Ladengriff_v3 (Autodesk Fusion 360 design; units mm, degrees)
Autodesk Fusion 360 part; units mm, degrees
sketch "Skizze1" plane through (0, 0, 0) normal (0, 1, 0) x (1, 0, 0)
  line L0 (0, 0) -> (7, 0)
  line L1 (7, 0) -> (7, 3.4)
  line L2 (0, 0) -> (0, 2.9)
  line L3 (7, 0) -> (7, 3.8137)
  line L4 (7, 3.8137) -> (4, 3.8137) construction
  line L5 (4, 3.8137) -> (4, 0)
  line L6 (4.4659, 0) -> (4.7043, 0)
  arc A0 (7, 3.4) -> (0, 2.9) centre (4.161, -6.1039) ccw
  line L7 (0, 2.9) -> (-13.5, 5)
  line L8 (0, 0) -> (0, -2.9)
  line L9 (0, -2.9) -> (-13.5, -5)
  line L10 (4.4659, 0) -> (4.7043, 0)
  line L11 (7, -3.8137) -> (4, -3.8137) construction
  arc A1 (0, -2.9) -> (7, -3.4) centre (4.161, 6.1039) ccw
  line L12 (0, 0) -> (7, 0)
  line L13 (4, -3.8137) -> (4, 0)
  line L14 (7, 0) -> (7, -3.4)
  line L15 (7, 0) -> (7, -3.8137)
  circle A2 centre (4.6733, 0) radius 5.5 construction
  arc A3 (7, 3) -> (0, 2.8) centre (3.7841, -7.0451) ccw
  line L16 (-0.4, 4.5) -> (-0.4, -4.248)
  circle A4 centre (4.4696, 0) radius 5.65 construction
  line L17 (10.1196, 2.0816) -> (10.1196, -2.0184)
  line L18 (9.7196, 2.7) -> (9.7196, -3.1376)
  line L19 (-1.1804, -2.5) -> (-1.1804, 3.5) construction
  circle A5 centre (8.1317, 0) radius 9
  line L20 (16.6917, -5.0993) -> (16.6917, 5.4007)
  dimension "d1" = 7
  dimension "d2" = 3.4
  dimension "d3" = 2.9
  dimension "d7" = 3
  dimension "d8" = 5
  dimension "d9" = 20.5
  dimension "d10" = 11
  dimension "d11" = 0.4
  dimension "d12" = 11.3
  dimension "d21" = 0.4
  dimension "d30" = 18
  constraint coincident L0.start L2.start
  constraint horizontal L0
  constraint perpendicular L0 L1
  constraint perpendicular L0 L2
  constraint perpendicular L0 L3
  constraint perpendicular L1 L4
  constraint coincident L0 L5.end
  constraint perpendicular L0 L5
  constraint coincident L0 L6.start
  constraint coincident L4.end A0
  constraint symmetric L2.start L0 L8.start
  constraint symmetric L1.start L0 L3.start
  constraint symmetric L0 L1.end A1.end
  constraint symmetric L0 L2.start L8.start
  constraint symmetric L0 L2.end L8.end
  constraint symmetric L0 L3.end L11.start
  constraint symmetric L0 L4.end L11.end
  constraint symmetric L0 L5.end L13.end
  constraint symmetric L0 L6.start L10.start
  constraint symmetric L0 L6.end L10.end
  constraint symmetric L0 A0 A1
  constraint symmetric L0 L7.end L9.end
  constraint coincident L2.end A2
  constraint coincident L8.end A2
  constraint vertical L16
  constraint vertical L17
  constraint tangent A4 L17
  constraint vertical L18
  constraint vertical L19
  constraint tangent A4 L19
  constraint vertical L20
  measures "d1" distance of L0.start L0.end
  measures "d2" distance of L0.end L1.end
  measures "d3" distance of L0.start L2.end
  measures "d7" distance of L3.end L4.end
  measures "d8" vertical distance of L0.start L7.end
  measures "d9" horizontal distance of L0.end L7.end
  measures "d10" diameter of A2
  measures "d11" distance of L2 L16
  measures "d12" diameter of A4
  measures "d21" distance of L17 L18
  measures "d30" diameter of A5
extrude "Extrusion1" add sketch "Skizze1" along normal blind 187 contours L1 L3 A0 L7 L9 A1 L14 L15 A5 L20 makes body 1
fillet "Abrundung1" radius 0.5 8 edges at (3.4543, 187, -3.7898) (7, 187, 0) (3.4543, 187, 3.7898) (-0.1843, 187, 2.9287) (-0.1843, 0, -2.9287) (-0.1843, 0, 2.9287) (3.4543, 0, -3.7898) (-0.1843, 187, -2.9287) on bodies 1
fillet "Abrundung1" radius 1.5 8 edges at (8.2255, 187, 8.9995) (16.6917, 187, 0) (8.2255, 187, -8.9995) (8.2255, 0, 8.9995) (16.6917, 0, 0) (8.2255, 0, -8.9995) (16.6917, 93.5, 2.7797) (16.6917, 93.5, -2.7797) on bodies 1
fillet "Abrundung2" radius 0.15 6 edges at (-0.2727, 0.9742, -2.9424) (-0.3685, 93.5, -2.9573) (-0.2727, 186.0258, -2.9424) (-0.2727, 0.9742, 2.9424) (-0.3685, 93.5, 2.9573) (-0.2727, 186.0258, 2.9424) on bodies 1
ref_plane "Arbeitsebene1" through (0, 2, 0) normal (0, 1, 0) x (0, 0, 1)
ref_plane "Arbeitsebene2" through (0, 185, 0) normal (0, 1, 0) x (0, 0, 1)
sphere "Grundkörper Kugel3" add diameter 1.1 placed x (1, 0, 0) y (0, 0, -1) z (0, 1, 0) at (0, 2, 3) separate body makes body 2
sphere "Grundkörper Kugel4" add diameter 1.1 placed x (1, 0, 0) y (0, 0, -1) z (0, 1, 0) at (0, 185, 3) separate body makes body 3
move_body "Fläche verschieben2" bodies 3 to x (1, 0, 0) y (0, 1, 0) z (0, 0, 1) at (0, 0, -0.11) on bodies 3
move_body "Fläche verschieben3" bodies 2 to x (1, 0, 0) y (0, 1, 0) z (0, 0, 1) at (0, 0, -0.19) on bodies 2
equation "d2 = 3.4 mm + luft"
equation "d3 = 2.9 mm + luft"
equation "d13 = laenge_griff + 5 mm"
equation "d25 = laenge_griff + 5 mm - 2 mm"
equation "laenge_griff = 182 mm"
equation "luft = 0 mm"
